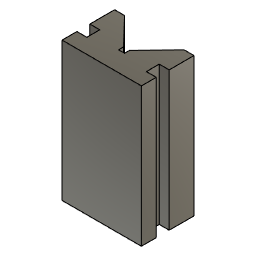
ex70 (Autodesk Fusion 360 design; units mm, degrees)
Autodesk Fusion 360 part; units mm, degrees
sketch "Sketch1" plane through (0, 0, 0) normal (0, 0, 1) x (1, 0, 0)
  line L0 (30, 2.5) -> (30, 15.5)
  line L1 (30, 15.5) -> (40, 15.5)
  line L2 (40, 15.5) -> (40, 40.5)
  line L3 (40, 40.5) -> (30, 40.5)
  line L4 (30, 40.5) -> (30, 15.5)
  line L5 (40, 40.5) -> (40, 15.5)
  line L6 (30, 12.5) -> (3, 12.5)
  line L7 (3, 12.5) -> (3, 7.5)
  line L8 (30, 40.5) -> (3, 12.5)
  line L9 (3, 7.5) -> (0, 7.5)
  line L10 (-30, 15.5) -> (-40, 15.5)
  line L11 (-30, 12.5) -> (-3, 12.5)
  line L12 (-40, 15.5) -> (-40, 40.5)
  line L13 (-40, 40.5) -> (-30, 40.5)
  line L14 (-30, 40.5) -> (-30, 15.5)
  line L15 (-30, 40.5) -> (-3, 12.5)
  line L16 (-3, 7.5) -> (0, 7.5)
  line L17 (-40, 40.5) -> (-40, 15.5)
  line L18 (-3, 12.5) -> (-3, 7.5)
  line L19 (-30, 2.5) -> (-30, 15.5)
  line L20 (40, -12.5) -> (-40, -12.5)
  line L21 (-40, -12.5) -> (-40, 2.5)
  line L22 (-40, 2.5) -> (40, 2.5)
  line L23 (40, 2.5) -> (40, -12.5)
  point P0 (0, 12.5)
  point P1 (0, 43.67)
  dimension "d13" = 80
  dimension "d14" = 15
  constraint horizontal L1
  constraint vertical L2
  constraint horizontal L3
  constraint vertical L4
  constraint perpendicular L1 L5
  constraint perpendicular L5 L6
  constraint perpendicular L7 L9
  constraint coincident L0 L6.start
  constraint horizontal L20
  constraint perpendicular L20 L21
  constraint parallel L20 L22
  constraint parallel L21 L23
  measures "d13" distance of L21.end L22.end
  measures "d14" distance of L20.end L21.end
extrude "Extrude1" add sketch "Sketch1" along normal blind 140
